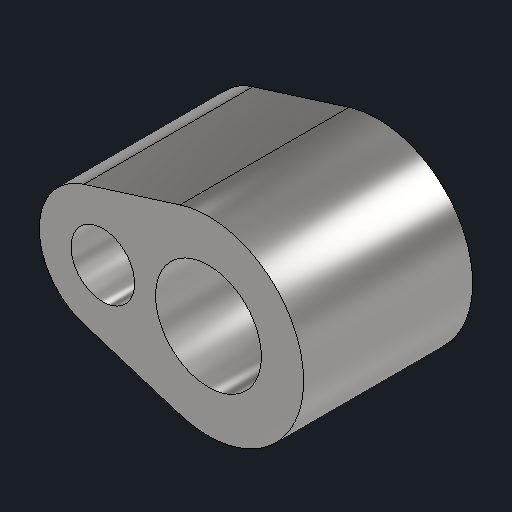
# Autodesk Inventor part: Anode Holding Nut
Saved by Autodesk Inventor 2027.1 (Build 311270010, 270A)
## iProperties
Created: 2024-05-17
Part Number: Anode Holding Nut
Material: Stainless Steel
Document SubType Name: Modeling
Designer: KAA
Density: 8 g/cm^3
Appearance: Semi-Polished
Author: KAA
Autodesk Inventor part; units mm, degrees
ref_plane "YZ Plane" through (0, 0, 0) normal (1, 0, 0) x (0, 1, 0)
ref_plane "XZ Plane" through (0, 0, 0) normal (0, 1, 0) x (-1, 0, 0)
ref_plane "XY Plane" through (0, 0, 0) normal (0, 0, 1) x (1, 0, 0)
sketch "Sketch1" plane through (0, 0, 0) normal (0, 0, 1) x (1, 0, 0)
  circle A0 centre (0, 0) radius 2.5
  circle A1 centre (-5, 0) radius 1.5
  arc A2 (-5.9, 2.8618) -> (-5.9, -2.8618) centre (-5, 0) ccw
  arc A3 (-1.35, -4.2927) -> (-1.35, 4.2927) centre (0, 0) ccw
  line L0 (-5.9, 2.8618) -> (-1.35, 4.2927)
  line L1 (-5.9, -2.8618) -> (-1.35, -4.2927)
  dimension "d0" = 5
  dimension "d1" = 3
  dimension "d2" = 9
  dimension "d3" = 5
  dimension "d4" = 1.5
  constraints: 5 point on circle, 4 centre point, 4 end point, 4 tangent, 3 coincident, 1 horizontal alignment
  measures "d0" diameter of A0
  measures "d1" diameter of A1
  measures "d2" diameter of A3
  measures "d3" distance of A1.centre point (0, 0)
  measures "d4" radial gap between concentric circles of A2 A1
extrude "Extrusion1" add sketch "Sketch1" along normal blind 8
sketch "Sketch2" plane through (0, 0, 0) normal (0, 0, -1) x (-1, 0, 0)
  circle A0 centre (5, 0) radius 1.5 projected
  circle A1 centre (5, 0) radius 1
  point P0 (0, 0)
  dimension "d21" = 2
  constraints: 1 centre point, 1 coincident
  measures "d21" diameter of A1
extrude "Extrusion2" add sketch "Sketch2" against normal blind 2
sketch "Sketch3" plane through (0, 0, 0) normal (1, 0, 0) x (0, 1, 0)
  circle A0 centre (0, 4) radius 1.5
  line L0 (2.5, 8) -> (2.5, 0) projected
  point P0 (0, 0)
  point P1 (2.5, 4)
  dimension "d13" = 3
  constraints: 1 centre point, 1 horizontal alignment, 1 midpoint, 1 vertical alignment
  measures "d13" diameter of A0
body "Solid1"
